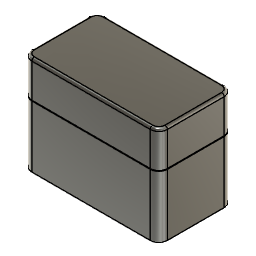
scatola (Autodesk Fusion 360 design; units mm, degrees)
Autodesk Fusion 360 part; units mm, degrees
sketch "Schizzo1" plane through (0, 0, 0) normal (0, 0, 1) x (1, 0, 0)
  line L0 (0, 0) -> (110, 0)
  line L1 (110, 0) -> (110, 60)
  line L2 (110, 60) -> (0, 60)
  line L3 (0, 60) -> (0, 0)
  dimension "d1" = 110
  dimension "d2" = 60
  constraint horizontal L0
  constraint vertical L1
  constraint horizontal L2
  constraint vertical L3
  constraint coincident L0.start L3.end
  measures "d1" distance of L0.start L0.end
  measures "d2" distance of L0.start L2.end
extrude "Estrusione1" add sketch "Schizzo1" along normal blind 80 makes body 1
fillet "Raccordo1" radius 7 4 edges at (110, 0, 40) (0, 0, 40) (110, 60, 40) (0, 60, 40) on bodies 1
ref_plane "Piano di lavoro1" through (55, 30, 55) normal (0, 0, 1) x (1, 0, 0)
split "Dividi1" by plane through (55, 30, 55) normal (0, 0, 1) bodies 1 makes body 2 at (71, 20, 80)
shell "Svuotamento1" thickness 4 removed faces 1 at (71, 20, 55) on bodies 1
shell "Svuotamento2" thickness 4 removed faces 1 at (71, 20, 55) on bodies 2
sketch "Schizzo2" plane through (0, 0, 55) normal (0, 0, 1) x (-1, 0, 0)
  arc A0 (-106, -53) -> (-103, -56) centre (-103, -53) ccw
  line L0 (-106, -53) -> (-106, -7)
  arc A1 (-103, -4) -> (-106, -7) centre (-103, -7) ccw
  line L1 (-103, -4) -> (-7, -4)
  arc A2 (-4, -7) -> (-7, -4) centre (-7, -7) ccw
  line L2 (-4, -7) -> (-4, -53)
  arc A3 (-7, -56) -> (-4, -53) centre (-7, -53) ccw
  line L3 (-7, -56) -> (-103, -56)
  arc A4 (0, -7) -> (-7, 0) centre (-7, -7) ccw
  line L4 (-7, 0) -> (-103, 0)
  arc A5 (-103, 0) -> (-110, -7) centre (-103, -7) ccw
  line L5 (-110, -7) -> (-110, -53)
  arc A6 (-110, -53) -> (-103, -60) centre (-103, -53) ccw
  line L6 (-103, -60) -> (-7, -60)
  arc A7 (-7, -60) -> (0, -53) centre (-7, -53) ccw
  line L7 (0, -53) -> (0, -7)
  arc A8 (-108, -53) -> (-103, -58) centre (-103, -53) ccw
  line L8 (-7, -58) -> (-103, -58)
  arc A9 (-7, -58) -> (-2, -53) centre (-7, -53) ccw
  line L9 (-2, -7) -> (-2, -53)
  arc A10 (-2, -7) -> (-7, -2) centre (-7, -7) ccw
  line L10 (-103, -2) -> (-7, -2)
  arc A11 (-103, -2) -> (-108, -7) centre (-103, -7) ccw
  line L11 (-108, -53) -> (-108, -7)
  arc A12 (-107, -53) -> (-103, -57) centre (-103, -53) ccw
  line L12 (-7, -57) -> (-103, -57)
  arc A13 (-7, -57) -> (-3, -53) centre (-7, -53) ccw
  line L13 (-3, -7) -> (-3, -53)
  arc A14 (-3, -7) -> (-7, -3) centre (-7, -7) ccw
  line L14 (-103, -3) -> (-7, -3)
  arc A15 (-103, -3) -> (-107, -7) centre (-103, -7) ccw
  line L15 (-107, -53) -> (-107, -7)
  dimension "d12" = -2
  dimension "d13" = -1
extrude "Estrusione6" add sketch "Schizzo2" against normal blind 5 contours A12 L12 A13 L13 A14 L14 A15 L15 bodies 2
extrude "Estrusione3" cut sketch "Schizzo2" against normal blind 5 contours A12 L12 A13 L13 A14 L14 A15 L15 bodies 1
extrude "Estrusione2" cut sketch "Schizzo2" against normal blind 5 contours A8 L8 A9 L9 A10 L10 A11 L11 | A12 L12 A13 L13 A14 L14 A15 L15 bodies 1
extrude "Estrusione4" add sketch "Schizzo2" against normal blind 5 contours A8 L8 A9 L9 A10 L10 A11 L11 bodies 1
extrude "Estrusione5" add sketch "Schizzo2" against normal blind 5 contours A4 L4 A5 L5 A6 L6 A7 L7 bodies 2
fillet "Raccordo2" radius 2 8 edges at (107.9497, 2.0503, 80) (110, 30, 80) (107.9497, 57.9497, 80) (55, 60, 80) (2.0503, 57.9497, 80) (0, 30, 80) (2.0503, 2.0503, 80) (55, 0, 80) on bodies 2
extrude "Estrusione7" cut 1 faces at (39, 1.3333, 50) along direction (0, 0, 1) blind 0.5 on bodies 2 bodies 2
ref_plane "Piano di lavoro2" through (55, 30, 27.5) normal (0, -1, 0) x (1, 0, 0)
sketch "Schizzo3" plane through (55, 30, 27.5) normal (0, -1, 0) x (1, 0, 0)
extrude "Estrusione8" cut sketch "Schizzo2" against normal blind 5 contours A4 L4 A5 L5 A6 L6 A7 L7 bodies 1
extrude "Estrusione9" add 1 faces at (39, 1.3333, 50.5) along direction (0, 0, -1) blind 2 on bodies 2 bodies 2
extrude "Estrusione10" cut 1 faces at (39, 1.3333, 48.5) along direction (0, 0, 1) blind 1 on bodies 2 bodies 2
extrude "Estrusione11" cut 1 faces at (39, 1.3333, 49.5) along direction (0, 0, 1) blind 1 on bodies 2 bodies 2
extrude "Estrusione12" cut 1 faces at (39, 57.6667, 55) along direction (0, 0, -1) blind 0.3 on bodies 1 bodies 1
extrude "Estrusione13" cut 1 faces at (71, 3.3333, 50) along direction (0, 0, 1) blind 0.2 on bodies 2 bodies 2
equation "parete = 4 mm"
equation "d9 = parete"
equation "d10 = parete"
equation "tolleranza = 1 mm"
equation "d12 = -parete / 2"
equation "d13 = d12 + tolleranza"
named bodies: "tappo"
